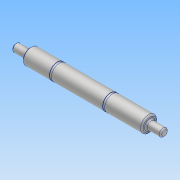
# Autodesk Inventor part: Top_Separator Shaft
Saved by Autodesk Inventor 2018.1 (Build 221171000, 171)
## iProperties
Created: 2019-02-27
Part Number: Top_Separator Shaft
Material: Aluminum 6061
Document SubType Name: Modeling
Designer: James
Density: 2.7 g/cm^3
Appearance: Aluminum - Flat
Author: James
Autodesk Inventor part; units mm, degrees
ref_plane "YZ Plane" through (0, 0, 0) normal (1, 0, 0) x (0, 1, 0)
ref_plane "XZ Plane" through (0, 0, 0) normal (0, 1, 0) x (-1, 0, 0)
ref_plane "XY Plane" through (0, 0, 0) normal (0, 0, 1) x (1, 0, 0)
sketch "Sketch1" plane through (0, 0, 0) normal (0, 0, 1) x (1, 0, 0)
  line L0 (0, 0) -> (45, 0)
  line L1 (45, 0) -> (45, 3)
  line L2 (45, 3) -> (0, 3)
  line L3 (0, 3) -> (0, 0)
  line L4 (0, 0) -> (-5.5, 0)
  line L5 (-5.5, 0) -> (-5.5, 1.5)
  line L6 (-5.5, 1.5) -> (0, 1.5)
  line L7 (0, 1.5) -> (0, 0)
  line L8 (45, 0) -> (50.5, 0)
  line L9 (50.5, 0) -> (50.5, 1.5)
  line L10 (50.5, 1.5) -> (45, 1.5)
  line L11 (45, 1.5) -> (45, 0)
  dimension "d0" = 3
  dimension "d1" = 45
  dimension "d2" = 1.5
  dimension "d3" = 5.5
  dimension "d4" = 1.5
  dimension "d5" = 5.5
  constraints: 24 end point, 6 parallel, 3 horizontal, 3 perpendicular
  measures "d0" distance of L0.end L1.end
  measures "d1" distance of L1.end L2.end
  measures "d2" distance of L4.end L5.end
  measures "d3" distance of L5.end L6.end
  measures "d4" distance of L8.end L9.end
  measures "d5" distance of L9.end L10.end
revolve "Revolution1" add sketch "Sketch1" angle 360 about axis through (0, 0, 0) along (1, 0, 0)
fillet "Fillet1" radius 0.5 2 edges at (45, -1.5, 0) (0, -1.5, 0)
chamfer "Chamfer1" distance 0.5 angle 45 4 edges at (-5.5, -1.5, 0) (0, -3, 0) (45, -3, 0) (50.5, -1.5, 0)
sketch "Sketch2" plane through (0, 0, 0) normal (0, 1, 0) x (-1, 0, 0)
  line L0 (-10.2, 3) -> (-11, 3)
  line L1 (-11, 3) -> (-11, 2.85)
  line L2 (-11, 2.85) -> (-10.2, 2.85)
  line L3 (-10.2, 2.85) -> (-10.2, 3)
  line L4 (-0.5, -3) -> (-0.5, 3) projected
  line L5 (-44.5, 3) -> (-44.5, -3) projected
  line L6 (6.7, 0) -> (-40.2, 0) projected
  line L7 (0, 2.5) -> (0, -2.5) projected
  line L8 (-30.2, 3) -> (-31, 3)
  line L9 (-31, 3) -> (-31, 2.85)
  line L10 (-31, 2.85) -> (-30.2, 2.85)
  line L11 (-30.2, 2.85) -> (-30.2, 3)
  line L12 (-45, -2.5) -> (-45, 2.5) projected
  point P0 (0, 0)
  dimension "d11" = 2.85
  dimension "d12" = 0.8
  dimension "d15" = 0.8
  dimension "d17" = 20
  dimension "d19" = 14
  dimension "d20" = 11
  constraints: 16 end point, 4 parallel, 3 horizontal alignment, 2 horizontal, 2 perpendicular
  measures "d11" distance between parallel lines of L6 L2
  measures "d12" distance of L0.start L0.end
  measures "d15" distance of L8.start L8.end
  measures "d17" distance of L9.end L1.end
  measures "d19" horizontal distance of L8.end L12.end
  measures "d20" distance from line of L0.end L7
revolve "Revolution2" cut sketch "Sketch2" angle 360 about axis through (-10, 0, 0) along (1, 0, 0)
equation "\"d4\" = d2"
equation "\"d15\" = d12"
body "Solid1"
